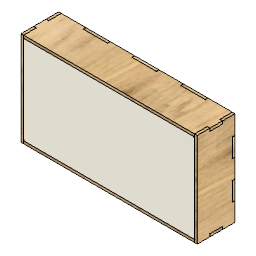
Cronus (Autodesk Fusion 360 design; units mm, degrees)
Autodesk Fusion 360 part; units mm, degrees
note: some values were not read from the file. Set by a fixed rule: which face or edge a step refers to.
(part 1 of 2)
sketch "Sketch1" plane through (0, 0, 0) normal (0, 1, 0) x (1, 0, 0) in component "Display"
  line L0 (0, 0) -> (65.5, 0)
  line L1 (65.5, 0) -> (65.5, -66.5)
  line L2 (65.5, -66.5) -> (0, -66.5)
  line L3 (0, -66.5) -> (0, 0)
  line L4 (0, -66.5) -> (1.55, -66.5) construction
  line L5 (1.55, -66.5) -> (1.55, -65.85) construction
  line L6 (1.55, -65.85) -> (6.55, -65.85)
  line L7 (6.55, -65.85) -> (6.55, -60.85)
  line L8 (6.55, -60.85) -> (1.55, -60.85)
  line L9 (1.55, -60.85) -> (1.55, -65.85)
  line L10 (14.75, -60.85) -> (9.75, -60.85)
  line L11 (9.75, -60.85) -> (9.75, -65.85)
  line L12 (9.75, -65.85) -> (14.75, -65.85)
  line L13 (14.75, -65.85) -> (14.75, -60.85)
  line L14 (22.95, -60.85) -> (17.95, -60.85)
  line L15 (17.95, -60.85) -> (17.95, -65.85)
  line L16 (17.95, -65.85) -> (22.95, -65.85)
  line L17 (22.95, -65.85) -> (22.95, -60.85)
  line L18 (31.15, -60.85) -> (26.15, -60.85)
  line L19 (26.15, -60.85) -> (26.15, -65.85)
  line L20 (26.15, -65.85) -> (31.15, -65.85)
  line L21 (31.15, -65.85) -> (31.15, -60.85)
  line L22 (39.35, -60.85) -> (34.35, -60.85)
  line L23 (34.35, -60.85) -> (34.35, -65.85)
  line L24 (34.35, -65.85) -> (39.35, -65.85)
  line L25 (39.35, -65.85) -> (39.35, -60.85)
  line L26 (47.55, -60.85) -> (42.55, -60.85)
  line L27 (42.55, -60.85) -> (42.55, -65.85)
  line L28 (42.55, -65.85) -> (47.55, -65.85)
  line L29 (47.55, -65.85) -> (47.55, -60.85)
  line L30 (55.75, -60.85) -> (50.75, -60.85)
  line L31 (50.75, -60.85) -> (50.75, -65.85)
  line L32 (50.75, -65.85) -> (55.75, -65.85)
  line L33 (55.75, -65.85) -> (55.75, -60.85)
  line L34 (63.95, -60.85) -> (58.95, -60.85)
  line L35 (58.95, -60.85) -> (58.95, -65.85)
  line L36 (58.95, -65.85) -> (63.95, -65.85)
  line L37 (63.95, -65.85) -> (63.95, -60.85)
  line L38 (6.55, -52.25) -> (1.55, -52.25)
  line L39 (1.55, -52.25) -> (1.55, -57.25)
  line L40 (1.55, -57.25) -> (6.55, -57.25)
  line L41 (6.55, -57.25) -> (6.55, -52.25)
  line L42 (14.75, -52.25) -> (9.75, -52.25)
  line L43 (9.75, -52.25) -> (9.75, -57.25)
  line L44 (9.75, -57.25) -> (14.75, -57.25)
  line L45 (14.75, -57.25) -> (14.75, -52.25)
  line L46 (22.95, -52.25) -> (17.95, -52.25)
  line L47 (17.95, -52.25) -> (17.95, -57.25)
  line L48 (17.95, -57.25) -> (22.95, -57.25)
  line L49 (22.95, -57.25) -> (22.95, -52.25)
  line L50 (31.15, -52.25) -> (26.15, -52.25)
  line L51 (26.15, -52.25) -> (26.15, -57.25)
  line L52 (26.15, -57.25) -> (31.15, -57.25)
  line L53 (31.15, -57.25) -> (31.15, -52.25)
  line L54 (39.35, -52.25) -> (34.35, -52.25)
  line L55 (34.35, -52.25) -> (34.35, -57.25)
  line L56 (34.35, -57.25) -> (39.35, -57.25)
  line L57 (39.35, -57.25) -> (39.35, -52.25)
  line L58 (47.55, -52.25) -> (42.55, -52.25)
  line L59 (42.55, -52.25) -> (42.55, -57.25)
  line L60 (42.55, -57.25) -> (47.55, -57.25)
  line L61 (47.55, -57.25) -> (47.55, -52.25)
  line L62 (55.75, -52.25) -> (50.75, -52.25)
  line L63 (50.75, -52.25) -> (50.75, -57.25)
  line L64 (50.75, -57.25) -> (55.75, -57.25)
  line L65 (55.75, -57.25) -> (55.75, -52.25)
  line L66 (63.95, -52.25) -> (58.95, -52.25)
  line L67 (58.95, -52.25) -> (58.95, -57.25)
  line L68 (58.95, -57.25) -> (63.95, -57.25)
  line L69 (63.95, -57.25) -> (63.95, -52.25)
  line L70 (6.55, -43.65) -> (1.55, -43.65)
  line L71 (1.55, -43.65) -> (1.55, -48.65)
  line L72 (1.55, -48.65) -> (6.55, -48.65)
  line L73 (6.55, -48.65) -> (6.55, -43.65)
  line L74 (14.75, -43.65) -> (9.75, -43.65)
  line L75 (9.75, -43.65) -> (9.75, -48.65)
  line L76 (9.75, -48.65) -> (14.75, -48.65)
  line L77 (14.75, -48.65) -> (14.75, -43.65)
  line L78 (22.95, -43.65) -> (17.95, -43.65)
  line L79 (17.95, -43.65) -> (17.95, -48.65)
  line L80 (17.95, -48.65) -> (22.95, -48.65)
  line L81 (22.95, -48.65) -> (22.95, -43.65)
  line L82 (31.15, -43.65) -> (26.15, -43.65)
  line L83 (26.15, -43.65) -> (26.15, -48.65)
  line L84 (26.15, -48.65) -> (31.15, -48.65)
  line L85 (31.15, -48.65) -> (31.15, -43.65)
  line L86 (39.35, -43.65) -> (34.35, -43.65)
  line L87 (34.35, -43.65) -> (34.35, -48.65)
  line L88 (34.35, -48.65) -> (39.35, -48.65)
  line L89 (39.35, -48.65) -> (39.35, -43.65)
  line L90 (47.55, -43.65) -> (42.55, -43.65)
  line L91 (42.55, -43.65) -> (42.55, -48.65)
  line L92 (42.55, -48.65) -> (47.55, -48.65)
  line L93 (47.55, -48.65) -> (47.55, -43.65)
  line L94 (55.75, -43.65) -> (50.75, -43.65)
  line L95 (50.75, -43.65) -> (50.75, -48.65)
  line L96 (50.75, -48.65) -> (55.75, -48.65)
  line L97 (55.75, -48.65) -> (55.75, -43.65)
  line L98 (63.95, -43.65) -> (58.95, -43.65)
  line L99 (58.95, -43.65) -> (58.95, -48.65)
  line L100 (58.95, -48.65) -> (63.95, -48.65)
  line L101 (63.95, -48.65) -> (63.95, -43.65)
  line L102 (6.55, -35.05) -> (1.55, -35.05)
  line L103 (1.55, -35.05) -> (1.55, -40.05)
  line L104 (1.55, -40.05) -> (6.55, -40.05)
  line L105 (6.55, -40.05) -> (6.55, -35.05)
  line L106 (14.75, -35.05) -> (9.75, -35.05)
  line L107 (9.75, -35.05) -> (9.75, -40.05)
  line L108 (9.75, -40.05) -> (14.75, -40.05)
  line L109 (14.75, -40.05) -> (14.75, -35.05)
  line L110 (22.95, -35.05) -> (17.95, -35.05)
  line L111 (17.95, -35.05) -> (17.95, -40.05)
  line L112 (17.95, -40.05) -> (22.95, -40.05)
  line L113 (22.95, -40.05) -> (22.95, -35.05)
  line L114 (31.15, -35.05) -> (26.15, -35.05)
  line L115 (26.15, -35.05) -> (26.15, -40.05)
  line L116 (26.15, -40.05) -> (31.15, -40.05)
  line L117 (31.15, -40.05) -> (31.15, -35.05)
  line L118 (39.35, -35.05) -> (34.35, -35.05)
  line L119 (34.35, -35.05) -> (34.35, -40.05)
  line L120 (34.35, -40.05) -> (39.35, -40.05)
  line L121 (39.35, -40.05) -> (39.35, -35.05)
  line L122 (47.55, -35.05) -> (42.55, -35.05)
  line L123 (42.55, -35.05) -> (42.55, -40.05)
  line L124 (42.55, -40.05) -> (47.55, -40.05)
  line L125 (47.55, -40.05) -> (47.55, -35.05)
  line L126 (55.75, -35.05) -> (50.75, -35.05)
  line L127 (50.75, -35.05) -> (50.75, -40.05)
  line L128 (50.75, -40.05) -> (55.75, -40.05)
  line L129 (55.75, -40.05) -> (55.75, -35.05)
  line L130 (63.95, -35.05) -> (58.95, -35.05)
  line L131 (58.95, -35.05) -> (58.95, -40.05)
  line L132 (58.95, -40.05) -> (63.95, -40.05)
  line L133 (63.95, -40.05) -> (63.95, -35.05)
  line L134 (6.55, -26.45) -> (1.55, -26.45)
  line L135 (1.55, -26.45) -> (1.55, -31.45)
  line L136 (1.55, -31.45) -> (6.55, -31.45)
  line L137 (6.55, -31.45) -> (6.55, -26.45)
  line L138 (14.75, -26.45) -> (9.75, -26.45)
  line L139 (9.75, -26.45) -> (9.75, -31.45)
  line L140 (9.75, -31.45) -> (14.75, -31.45)
  line L141 (14.75, -31.45) -> (14.75, -26.45)
  line L142 (22.95, -26.45) -> (17.95, -26.45)
  line L143 (17.95, -26.45) -> (17.95, -31.45)
  line L144 (17.95, -31.45) -> (22.95, -31.45)
  line L145 (22.95, -31.45) -> (22.95, -26.45)
  line L146 (31.15, -26.45) -> (26.15, -26.45)
  line L147 (26.15, -26.45) -> (26.15, -31.45)
  line L148 (26.15, -31.45) -> (31.15, -31.45)
  line L149 (31.15, -31.45) -> (31.15, -26.45)
  line L150 (39.35, -26.45) -> (34.35, -26.45)
  line L151 (34.35, -26.45) -> (34.35, -31.45)
  line L152 (34.35, -31.45) -> (39.35, -31.45)
  line L153 (39.35, -31.45) -> (39.35, -26.45)
  line L154 (47.55, -26.45) -> (42.55, -26.45)
  line L155 (42.55, -26.45) -> (42.55, -31.45)
  line L156 (42.55, -31.45) -> (47.55, -31.45)
  line L157 (47.55, -31.45) -> (47.55, -26.45)
  line L158 (55.75, -26.45) -> (50.75, -26.45)
  line L159 (50.75, -26.45) -> (50.75, -31.45)
  line L160 (50.75, -31.45) -> (55.75, -31.45)
  line L161 (55.75, -31.45) -> (55.75, -26.45)
  line L162 (63.95, -26.45) -> (58.95, -26.45)
  line L163 (58.95, -26.45) -> (58.95, -31.45)
  line L164 (58.95, -31.45) -> (63.95, -31.45)
  line L165 (63.95, -31.45) -> (63.95, -26.45)
  line L166 (6.55, -17.85) -> (1.55, -17.85)
  line L167 (1.55, -17.85) -> (1.55, -22.85)
  line L168 (1.55, -22.85) -> (6.55, -22.85)
  line L169 (6.55, -22.85) -> (6.55, -17.85)
  line L170 (14.75, -17.85) -> (9.75, -17.85)
  line L171 (9.75, -17.85) -> (9.75, -22.85)
  line L172 (9.75, -22.85) -> (14.75, -22.85)
  line L173 (14.75, -22.85) -> (14.75, -17.85)
  line L174 (22.95, -17.85) -> (17.95, -17.85)
  line L175 (17.95, -17.85) -> (17.95, -22.85)
  line L176 (17.95, -22.85) -> (22.95, -22.85)
  line L177 (22.95, -22.85) -> (22.95, -17.85)
  line L178 (31.15, -17.85) -> (26.15, -17.85)
  line L179 (26.15, -17.85) -> (26.15, -22.85)
  line L180 (26.15, -22.85) -> (31.15, -22.85)
  line L181 (31.15, -22.85) -> (31.15, -17.85)
  line L182 (39.35, -17.85) -> (34.35, -17.85)
  line L183 (34.35, -17.85) -> (34.35, -22.85)
  line L184 (34.35, -22.85) -> (39.35, -22.85)
  line L185 (39.35, -22.85) -> (39.35, -17.85)
  line L186 (47.55, -17.85) -> (42.55, -17.85)
  line L187 (42.55, -17.85) -> (42.55, -22.85)
  line L188 (42.55, -22.85) -> (47.55, -22.85)
  line L189 (47.55, -22.85) -> (47.55, -17.85)
  line L190 (55.75, -17.85) -> (50.75, -17.85)
  line L191 (50.75, -17.85) -> (50.75, -22.85)
  line L192 (50.75, -22.85) -> (55.75, -22.85)
  line L193 (55.75, -22.85) -> (55.75, -17.85)
  line L194 (63.95, -17.85) -> (58.95, -17.85)
  line L195 (58.95, -17.85) -> (58.95, -22.85)
  line L196 (58.95, -22.85) -> (63.95, -22.85)
  line L197 (63.95, -22.85) -> (63.95, -17.85)
  line L198 (6.55, -9.25) -> (1.55, -9.25)
  line L199 (1.55, -9.25) -> (1.55, -14.25)
  line L200 (1.55, -14.25) -> (6.55, -14.25)
  line L201 (6.55, -14.25) -> (6.55, -9.25)
  line L202 (14.75, -9.25) -> (9.75, -9.25)
  line L203 (9.75, -9.25) -> (9.75, -14.25)
  line L204 (9.75, -14.25) -> (14.75, -14.25)
  line L205 (14.75, -14.25) -> (14.75, -9.25)
  line L206 (22.95, -9.25) -> (17.95, -9.25)
  line L207 (17.95, -9.25) -> (17.95, -14.25)
  line L208 (17.95, -14.25) -> (22.95, -14.25)
  line L209 (22.95, -14.25) -> (22.95, -9.25)
  line L210 (31.15, -9.25) -> (26.15, -9.25)
  line L211 (26.15, -9.25) -> (26.15, -14.25)
  line L212 (26.15, -14.25) -> (31.15, -14.25)
  line L213 (31.15, -14.25) -> (31.15, -9.25)
  line L214 (39.35, -9.25) -> (34.35, -9.25)
  line L215 (34.35, -9.25) -> (34.35, -14.25)
  line L216 (34.35, -14.25) -> (39.35, -14.25)
  line L217 (39.35, -14.25) -> (39.35, -9.25)
  line L218 (47.55, -9.25) -> (42.55, -9.25)
  line L219 (42.55, -9.25) -> (42.55, -14.25)
  line L220 (42.55, -14.25) -> (47.55, -14.25)
  line L221 (47.55, -14.25) -> (47.55, -9.25)
  line L222 (55.75, -9.25) -> (50.75, -9.25)
  line L223 (50.75, -9.25) -> (50.75, -14.25)
  line L224 (50.75, -14.25) -> (55.75, -14.25)
  line L225 (55.75, -14.25) -> (55.75, -9.25)
  line L226 (63.95, -9.25) -> (58.95, -9.25)
  line L227 (58.95, -9.25) -> (58.95, -14.25)
  line L228 (58.95, -14.25) -> (63.95, -14.25)
  line L229 (63.95, -14.25) -> (63.95, -9.25)
  line L230 (6.55, -0.65) -> (1.55, -0.65)
  line L231 (1.55, -0.65) -> (1.55, -5.65)
  line L232 (1.55, -5.65) -> (6.55, -5.65)
  line L233 (6.55, -5.65) -> (6.55, -0.65)
  line L234 (14.75, -0.65) -> (9.75, -0.65)
  line L235 (9.75, -0.65) -> (9.75, -5.65)
  line L236 (9.75, -5.65) -> (14.75, -5.65)
  line L237 (14.75, -5.65) -> (14.75, -0.65)
  line L238 (22.95, -0.65) -> (17.95, -0.65)
  line L239 (17.95, -0.65) -> (17.95, -5.65)
  line L240 (17.95, -5.65) -> (22.95, -5.65)
  line L241 (22.95, -5.65) -> (22.95, -0.65)
  line L242 (31.15, -0.65) -> (26.15, -0.65)
  line L243 (26.15, -0.65) -> (26.15, -5.65)
  line L244 (26.15, -5.65) -> (31.15, -5.65)
  line L245 (31.15, -5.65) -> (31.15, -0.65)
  line L246 (39.35, -0.65) -> (34.35, -0.65)
  line L247 (34.35, -0.65) -> (34.35, -5.65)
  line L248 (34.35, -5.65) -> (39.35, -5.65)
  line L249 (39.35, -5.65) -> (39.35, -0.65)
  line L250 (47.55, -0.65) -> (42.55, -0.65)
  line L251 (42.55, -0.65) -> (42.55, -5.65)
  line L252 (42.55, -5.65) -> (47.55, -5.65)
  line L253 (47.55, -5.65) -> (47.55, -0.65)
  line L254 (55.75, -0.65) -> (50.75, -0.65)
  line L255 (50.75, -0.65) -> (50.75, -5.65)
  line L256 (50.75, -5.65) -> (55.75, -5.65)
  line L257 (55.75, -5.65) -> (55.75, -0.65)
  line L258 (63.95, -0.65) -> (58.95, -0.65)
  line L259 (58.95, -0.65) -> (58.95, -5.65)
  line L260 (58.95, -5.65) -> (63.95, -5.65)
  line L261 (63.95, -5.65) -> (63.95, -0.65)
  line L262 (0, -66.5) -> (1.45, -66.5) construction
  line L263 (32.75, -66.5) -> (32.75, 0) construction
  line L264 (0, -66.5) -> (8, -66.5) construction
  line L265 (8, -66.5) -> (8, 0) construction
  circle A0 centre (8, -33.25) radius 0.95
  circle A1 centre (8, -58.75) radius 0.95 construction
  circle A2 centre (8, -7.75) radius 0.95
  circle A3 centre (57.5, -58.75) radius 0.95
  circle A4 centre (57.5, -33.25) radius 0.95
  circle A5 centre (57.5, -7.75) radius 0.95 construction
  line L266 (0, -66.5) -> (9, -66.5)
  line L267 (9, -66.5) -> (9, -60.85)
  line L268 (9, -60.85) -> (0, -60.85)
  line L269 (0, -60.85) -> (0, -66.5)
  line L270 (65.5, 0) -> (57.5, 0)
  line L271 (56.25, 0) -> (56.25, -5.65)
  line L272 (56.25, -5.65) -> (65.5, -5.65)
  line L273 (65.5, -5.65) -> (65.5, 0)
  dimension "d3" = 65.5
  dimension "d4" = 66.5
  dimension "d5" = 1.55
  dimension "d6" = 0.65
  dimension "d7" = 5
  dimension "d8" = 5
  dimension "d11" = 8.2
  dimension "d12" = 8.6
  dimension "d256" = 8
  dimension "d257" = 1.9
  dimension "d260" = 0
  dimension "d261" = 25.5
  dimension "d276" = 1
  dimension "d277" = 0.5
  constraint horizontal L0
  constraint vertical L1
  constraint horizontal L2
  constraint vertical L3
  constraint coincident L0.start L3.end
  constraint perpendicular L3 L4
  constraint vertical L5
  constraint horizontal L6
  constraint vertical L7
  constraint horizontal L8
  constraint vertical L9
  constraint horizontal L262
  constraint midpoint L2 L263.start
  constraint midpoint L0 L263.end
  constraint horizontal L264
  constraint coincident L0 L265.end
  constraint perpendicular L0 L265
  constraint midpoint L265 A0.centre
  constraint symmetric L263 A0 A4
  constraint symmetric L263 A1 A3
  constraint symmetric L263 A2 A5
  constraint horizontal L266
  constraint vertical L267
  constraint horizontal L268
  constraint vertical L269
  constraint collinear L8 L268
  constraint horizontal L270
  constraint vertical L271
  constraint horizontal L272
  constraint vertical L273
  constraint coincident L271.end L272.start
  constraint coincident L0 L271.start
  constraint collinear L260 L272
  measures "d3" distance of L0.start L0.end
  measures "d4" distance of L0.start L2.end
  measures "d5" distance of L2.end L4.end
  measures "d6" distance of L4.end L5.end
  measures "d7" distance of L5.end L6.end
  measures "d8" distance of L5.end L8.end
  measures "d256" distance of L2.end L264.end
  measures "d257" diameter of A0
  measures "d276" distance of L265 L267
  measures "d277" distance of L257 L271
extrude "Extrude3" add sketch "Sketch1" against normal blind 1.4 contours L0 L1 L2 L3 L8 L260 L267 L268 L271 L272 | L10 L11 L12 L13 | L14 L15 L16 L17 | L18 L19 L20 L21 | L22 L23 L24 L25 | L26 L27 L28 L29 | L30 L31 L32 L33 | L34 L35 L36 L37 | L38 L39 L40 L41 | L42 L43 L44 L45 | L46 L47 L48 L49 | L50 L51 L52 L53 | L54 L55 L56 L57 | L58 L59 L60 L61 | L62 L63 L64 L65 | L66 L67 L68 L69 | L70 L71 L72 L73 | L74 L75 L76 L77 | L78 L79 L80 L81 | L82 L83 L84 L85 | L86 L87 L88 L89 | L90 L91 L92 L93 | L94 L95 L96 L97 | L98 L99 L100 L101 | L102 L103 L104 L105 | L106 L107 L108 L109 | L110 L111 L112 L113 | L114 L115 L116 L117 | L118 L119 L120 L121 | L122 L123 L124 L125 | L126 L127 L128 L129 | L130 L131 L132 L133 | L134 L135 L136 L137 | L138 L139 L140 L141 | L142 L143 L144 L145 | L146 L147 L148 L149 | L150 L151 L152 L153 | L154 L155 L156 L157 | L158 L159 L160 L161 | L162 L163 L164 L165 | L166 L167 L168 L169 | L170 L171 L172 L173 | L174 L175 L176 L177 | L178 L179 L180 L181 | L182 L183 L184 L185 | L186 L187 L188 L189 | L190 L191 L192 L193 | L194 L195 L196 L197 | L198 L199 L200 L201 | L202 L203 L204 L205 | L206 L207 L208 L209 | L210 L211 L212 L213 | L214 L215 L216 L217 | L218 L219 L220 L221 | L222 L223 L224 L225 | L226 L227 L228 L229 | L230 L231 L232 L233 | L234 L235 L236 L237 | L238 L239 L240 L241 | L242 L243 L244 L245 | L246 L247 L248 L249 | L250 L251 L252 L253 | L254 L255 L256 L257 makes body 1 in component "Display"
extrude "Extrude1" add sketch "Sketch1" against normal blind 3 contours L6 L7 L8 L9 L268 | L258 L259 L260 L261 L272 | L10 L11 L12 L13 | L14 L15 L16 L17 | L18 L19 L20 L21 | L22 L23 L24 L25 | L26 L27 L28 L29 | L30 L31 L32 L33 | L34 L35 L36 L37 | L38 L39 L40 L41 | L42 L43 L44 L45 | L46 L47 L48 L49 | L50 L51 L52 L53 | L54 L55 L56 L57 | L58 L59 L60 L61 | L62 L63 L64 L65 | L66 L67 L68 L69 | L70 L71 L72 L73 | L74 L75 L76 L77 | L78 L79 L80 L81 | L82 L83 L84 L85 | L86 L87 L88 L89 | L90 L91 L92 L93 | L94 L95 L96 L97 | L98 L99 L100 L101 | L102 L103 L104 L105 | L106 L107 L108 L109 | L110 L111 L112 L113 | L114 L115 L116 L117 | L118 L119 L120 L121 | L122 L123 L124 L125 | L126 L127 L128 L129 | L130 L131 L132 L133 | L134 L135 L136 L137 | L138 L139 L140 L141 | L142 L143 L144 L145 | L146 L147 L148 L149 | L150 L151 L152 L153 | L154 L155 L156 L157 | L158 L159 L160 L161 | L162 L163 L164 L165 | L166 L167 L168 L169 | L170 L171 L172 L173 | L174 L175 L176 L177 | L178 L179 L180 L181 | L182 L183 L184 L185 | L186 L187 L188 L189 | L190 L191 L192 L193 | L194 L195 L196 L197 | L198 L199 L200 L201 | L202 L203 L204 L205 | L206 L207 L208 L209 | L210 L211 L212 L213 | L214 L215 L216 L217 | L218 L219 L220 L221 | L222 L223 L224 L225 | L226 L227 L228 L229 | L230 L231 L232 L233 | L234 L235 L236 L237 | L238 L239 L240 L241 | L242 L243 L244 L245 | L246 L247 L248 L249 | L250 L251 L252 L253 | L254 L255 L256 L257 bodies 1 in component "Display"
pattern_linear "R-Pattern1" count 4 spacing 65.5 along (1, 0, 0) count 2 spacing 68.5 along (0, 0, 1) of bodies 1 makes body 2 at (90.3041, 0, 51.0047) makes body 3 at (155.8041, 0, 51.0047) makes body 4 at (221.3041, 0, 51.0047) makes body 5 at (24.8041, 0, 119.5047) makes body 6 at (90.3041, 0, 119.5047) makes body 7 at (155.8041, 0, 119.5047) makes body 8 at (221.3041, 0, 119.5047) in component "Display"
sketch "Sketch2" plane through (0, 0, 0) normal (0, 1, 0) x (1, 0, 0) in component "DisplayMount"
  line L0 (262, -135) -> (0, -135)
  line L1 (0, -135) -> (0, 0)
  line L2 (0, 0) -> (262, 0)
  line L3 (262, 0) -> (262, -135)
  line L4 (-1, -136) -> (-1, 1)
  line L5 (-1, 1) -> (263, 1)
  line L6 (263, 1) -> (263, -136)
  line L7 (263, -136) -> (-1, -136)
  point P0 (262, -135)
  constraint horizontal L0
  constraint vertical L1
  constraint horizontal L2
  constraint vertical L3
  constraint coincident L1.end L2.start
  constraint coincident P0 L0.start
extrude "Extrude2" add sketch "Sketch2" along normal blind 3 separate body contours L0 L1 L2 L3 | L4 L5 L6 L7 makes body 9 in component "DisplayMount"
sketch "Sketch3" plane through (0, 3, 0) normal (0, 1, 0) x (-1, 0, 0) in component "DisplayMount"
  line L0 (-263, 136) -> (-263, -1)
  line L1 (-263, -1) -> (1, -1)
  line L2 (1, -1) -> (1, 136)
  line L3 (1, 136) -> (-263, 136)
  circle A0 centre (-57.5, 101.75) radius 0.95
  circle A1 centre (-8, 101.75) radius 0.95
  circle A2 centre (-57.5, 33.25) radius 0.95
  circle A3 centre (-8, 33.25) radius 0.95
  line L4 (-9, 135) -> (0, 135)
  line L5 (0, 135) -> (0, 129.35)
  line L6 (0, 129.35) -> (-9, 129.35)
  line L7 (-9, 129.35) -> (-9, 135)
  line L8 (-65.5, 74.15) -> (-56.25, 74.15)
  line L9 (-56.25, 74.15) -> (-56.25, 68.5)
  line L10 (-56.25, 68.5) -> (-65.5, 68.5)
  line L11 (-65.5, 68.5) -> (-65.5, 74.15)
  line L12 (-9, 66.5) -> (0, 66.5)
  line L13 (0, 66.5) -> (0, 60.85)
  line L14 (0, 60.85) -> (-9, 60.85)
  line L15 (-9, 60.85) -> (-9, 66.5)
  line L16 (-65.5, 5.65) -> (-56.25, 5.65)
  line L17 (-56.25, 5.65) -> (-56.25, 0)
  line L18 (-56.25, 0) -> (-65.5, 0)
  line L19 (-65.5, 0) -> (-65.5, 5.65)
  point P0 (-9, 135)
  point P1 (0, 129.35)
  point P2 (-9, 66.5)
  point P3 (0, 60.85)
  point P4 (-65.5, 74.15)
  point P5 (-56.25, 68.5)
  point P6 (-65.5, 5.65)
  point P7 (-56.25, 0)
  constraint horizontal L4
  constraint vertical L5
  constraint horizontal L6
  constraint vertical L7
  constraint horizontal L8
  constraint vertical L9
  constraint horizontal L10
  constraint vertical L11
  constraint horizontal L12
  constraint vertical L13
  constraint horizontal L14
  constraint vertical L15
  constraint horizontal L16
  constraint vertical L17
  constraint horizontal L18
  constraint vertical L19
  constraint coincident P2 L12.start
  constraint coincident P3 L13.end
  constraint coincident P0 L4.start
  constraint coincident P1 L5.end
  constraint coincident P4 L8.start
  constraint coincident P5 L9.end
  constraint coincident P6 L16.start
  constraint coincident P7 L17.end
extrude "Extrude3'" cut sketch "Sketch3" against normal up to surface (3 mm away) contours A0 | A1 | A2 | A3 | L4 L5 L6 L7 | L8 L9 L10 L11 | L12 L13 L14 L15 | L16 L17 L18 L19 bodies 9 in component "DisplayMount"
pattern_linear "R-Pattern3" count 4 spacing 65.5 along (1, 0, 0) of "Extrude3'" in component "DisplayMount"
ref_plane "WorkPlane1" through (131, 10, 67.5) normal (0, 1, 0) x (0, 0, 1) in component "PowerSupply"
sketch "Sketch2 (2)" plane through (0, 10, 0) normal (0, 1, 0) x (1, 0, 0) in component "PowerSupply"
  line L0 (236, -116) -> (178, -116)
  line L1 (178, -116) -> (178, -31)
  line L2 (178, -31) -> (236, -31)
  line L3 (236, -31) -> (236, -116)
  line L4 (236, -116) -> (230, -116) construction
  line L5 (230, -116) -> (230, -113) construction
  circle A0 centre (230, -113) radius 1.25
  line L6 (230, -113) -> (183, -113) construction
  line L7 (183, -113) -> (183, -35) construction
  line L8 (183, -35) -> (230, -35) construction
  line L9 (230, -35) -> (230, -113) construction
  circle A1 centre (183, -35) radius 1.25
  line L10 (230, -113) -> (183, -113) construction
  line L11 (183, -113) -> (183, -35) construction
  line L12 (183, -35) -> (230, -35) construction
  line L13 (230, -35) -> (230, -113) construction
  line L14 (230, -113) -> (183, -113) construction
  line L15 (183, -113) -> (183, -35) construction
  line L16 (183, -35) -> (230, -35) construction
  line L17 (230, -35) -> (230, -113) construction
  circle A2 centre (183, -113) radius 1.25
  circle A3 centre (230, -35) radius 1.25
  dimension "d145" = 58
  dimension "d146" = 85
  dimension "d147" = 6
  dimension "d148" = 90
  dimension "d149" = 3
  dimension "d150" = 2.5
  dimension "d151" = 47
  dimension "d152" = 78
  dimension "d153" = 2.5
  dimension "d242" = 2.5
  dimension "d243" = 2.5
  constraint horizontal L0
  constraint vertical L1
  constraint horizontal L2
  constraint vertical L3
  constraint coincident L0 L4.end
  constraint coincident L5.end A0.centre
  constraint horizontal L6
  constraint vertical L7
  constraint horizontal L8
  constraint vertical L9
  constraint coincident L7.end L8.start
  constraint horizontal L10
  constraint vertical L11
  constraint horizontal L12
  constraint vertical L13
  constraint horizontal L14
  constraint vertical L15
  constraint horizontal L16
  constraint vertical L17
  constraint coincident L6.end L7.start
  constraint coincident L8.end L9.start
  measures "d145" distance of L0.start L0.end
  measures "d146" distance of L0.start L2.end
  measures "d147" distance of L0.start L4.end
  measures "d148" angle of L4 L5
  measures "d149" distance of L4.end L5.end
  measures "d150" diameter of A0
  measures "d151" distance of L5.end L6.end
  measures "d152" distance of L5.end L8.end
  measures "d153" diameter of A1
  measures "d242" diameter of A2
  measures "d243" diameter of A3
extrude "Extrude1'" add sketch "Sketch2 (2)" along normal blind 34 separate body makes body 10 in component "PowerSupply"
sketch "Sketch11" plane through (0, 3, 0) normal (0, 1, 0) x (-1, 0, 0) in component "DisplayMount"
  line L0 (1, 136) -> (-263, 136)
  line L1 (-263, 136) -> (-263, -1)
  line L2 (-263, -1) -> (1, -1)
  circle A0 centre (-230, 113) radius 1.25
  circle A1 centre (-183, 35) radius 1.25
  circle A2 centre (-230, 113) radius 3.5
  circle A3 centre (-183, 35) radius 3.5
  line L3 (1, -1) -> (1, 136)
  line L4 (-97.9526, 89.8787) -> (-31.9526, 89.8787) construction
  line L5 (-31.9526, 89.8787) -> (-31.9526, 43.8787) construction
  line L6 (-31.9526, 43.8787) -> (-97.9526, 43.8787) construction
  line L7 (-97.9526, 43.8787) -> (-97.9526, 89.8787) construction
  circle A4 centre (-97.9526, 89.8787) radius 1
  circle A5 centre (-31.9526, 89.8787) radius 1
  circle A6 centre (-97.9526, 43.8787) radius 1
  circle A7 centre (-31.9526, 43.8787) radius 1
  circle A8 centre (-97.9526, 89.8787) radius 2.5
  circle A9 centre (-31.9526, 89.8787) radius 2.5
  circle A10 centre (-31.9526, 43.8787) radius 2.5
  circle A11 centre (-97.9526, 43.8787) radius 2.5
  circle A12 centre (-183, 113) radius 1.25
  circle A13 centre (-230, 35) radius 1.25
  circle A14 centre (-183, 113) radius 3.5
  circle A15 centre (-230, 35) radius 3.5
  circle A16 centre (-254, 33.25) radius 0.95
  line L8 (-262, 68.5) -> (-262, 74.15)
  line L9 (-262, 74.15) -> (-252.75, 74.15)
  line L10 (-252.75, 74.15) -> (-252.75, 68.5)
  line L11 (-252.75, 68.5) -> (-262, 68.5)
  line L12 (-205.5, 129.35) -> (-205.5, 135)
  line L13 (-205.5, 135) -> (-196.5, 135)
  line L14 (-196.5, 135) -> (-196.5, 129.35)
  line L15 (-196.5, 129.35) -> (-205.5, 129.35)
  circle A17 centre (-204.5, 101.75) radius 0.95
  circle A18 centre (-204.5, 33.25) radius 0.95
  line L16 (-262, 0) -> (-262, 5.65)
  line L17 (-262, 5.65) -> (-252.75, 5.65)
  line L18 (-252.75, 5.65) -> (-252.75, 0)
  line L19 (-252.75, 0) -> (-262, 0)
  line L20 (-205.5, 60.85) -> (-205.5, 66.5)
  line L21 (-205.5, 66.5) -> (-196.5, 66.5)
  line L22 (-196.5, 66.5) -> (-196.5, 60.85)
  line L23 (-196.5, 60.85) -> (-205.5, 60.85)
  circle A19 centre (-254, 101.75) radius 0.95
  circle A20 centre (-188.5, 33.25) radius 0.95
  line L24 (-196.5, 68.5) -> (-196.5, 74.15)
  line L25 (-196.5, 74.15) -> (-187.25, 74.15)
  line L26 (-187.25, 74.15) -> (-187.25, 68.5)
  line L27 (-187.25, 68.5) -> (-196.5, 68.5)
  line L28 (-140, 129.35) -> (-140, 135)
  line L29 (-140, 135) -> (-131, 135)
  line L30 (-131, 135) -> (-131, 129.35)
  line L31 (-131, 129.35) -> (-140, 129.35)
  circle A21 centre (-139, 101.75) radius 0.95
  circle A22 centre (-139, 33.25) radius 0.95
  line L32 (-196.5, 0) -> (-196.5, 5.65)
  line L33 (-196.5, 5.65) -> (-187.25, 5.65)
  line L34 (-187.25, 5.65) -> (-187.25, 0)
  line L35 (-187.25, 0) -> (-196.5, 0)
  line L36 (-140, 60.85) -> (-140, 66.5)
  line L37 (-140, 66.5) -> (-131, 66.5)
  line L38 (-131, 66.5) -> (-131, 60.85)
  line L39 (-131, 60.85) -> (-140, 60.85)
  circle A23 centre (-188.5, 101.75) radius 0.95
  circle A24 centre (-123, 33.25) radius 0.95
  line L40 (-131, 68.5) -> (-131, 74.15)
  line L41 (-131, 74.15) -> (-121.75, 74.15)
  line L42 (-121.75, 74.15) -> (-121.75, 68.5)
  line L43 (-121.75, 68.5) -> (-131, 68.5)
  line L44 (-74.5, 129.35) -> (-74.5, 135)
  line L45 (-74.5, 135) -> (-65.5, 135)
  line L46 (-65.5, 135) -> (-65.5, 129.35)
  line L47 (-65.5, 129.35) -> (-74.5, 129.35)
  circle A25 centre (-73.5, 101.75) radius 0.95
  circle A26 centre (-73.5, 33.25) radius 0.95
  line L48 (-131, 0) -> (-131, 5.65)
  line L49 (-131, 5.65) -> (-121.75, 5.65)
  line L50 (-121.75, 5.65) -> (-121.75, 0)
  line L51 (-121.75, 0) -> (-131, 0)
  line L52 (-74.5, 60.85) -> (-74.5, 66.5)
  line L53 (-74.5, 66.5) -> (-65.5, 66.5)
  line L54 (-65.5, 66.5) -> (-65.5, 60.85)
  line L55 (-65.5, 60.85) -> (-74.5, 60.85)
  circle A27 centre (-123, 101.75) radius 0.95
  circle A28 centre (-57.5, 33.25) radius 0.95
  line L56 (-65.5, 68.5) -> (-65.5, 74.15)
  line L57 (-65.5, 74.15) -> (-56.25, 74.15)
  line L58 (-56.25, 74.15) -> (-56.25, 68.5)
  line L59 (-56.25, 68.5) -> (-65.5, 68.5)
  line L60 (-9, 129.35) -> (-9, 135)
  line L61 (-9, 135) -> (0, 135)
  line L62 (0, 135) -> (0, 129.35)
  line L63 (0, 129.35) -> (-9, 129.35)
  circle A29 centre (-8, 101.75) radius 0.95
  circle A30 centre (-8, 33.25) radius 0.95
  line L64 (-65.5, 0) -> (-65.5, 5.65)
  line L65 (-65.5, 5.65) -> (-56.25, 5.65)
  line L66 (-56.25, 5.65) -> (-56.25, 0)
  line L67 (-56.25, 0) -> (-65.5, 0)
  line L68 (-9, 60.85) -> (-9, 66.5)
  line L69 (-9, 66.5) -> (0, 66.5)
  line L70 (0, 66.5) -> (0, 60.85)
  line L71 (0, 60.85) -> (-9, 60.85)
  circle A31 centre (-57.5, 101.75) radius 0.95
  dimension "d156" = 7
  dimension "d157" = 7
  dimension "d166" = 66
  dimension "d167" = 46
  dimension "d168" = 2
  dimension "d169" = 2
  dimension "d170" = 2
  dimension "d171" = 2
  dimension "d172" = 5
  dimension "d173" = 5
  dimension "d174" = 5
  dimension "d175" = 5
  dimension "d244" = 7
  dimension "d245" = 7
  constraint concentric A0 A2
  constraint concentric A1 A3
  constraint horizontal L4
  constraint vertical L5
  constraint horizontal L6
  constraint vertical L7
  constraint coincident L4.start L7.end
  constraint coincident L4.end L5.start
  constraint coincident L6.end L7.start
  constraint coincident L5.end L6.start
  constraint concentric A4 A8
  constraint concentric A5 A9
  constraint concentric A7 A10
  constraint concentric A6 A11
  constraint concentric A12 A14
  constraint concentric A13 A15
  measures "d156" diameter of A2
  measures "d157" diameter of A3
  measures "d166" distance of L4.start L4.end
  measures "d167" distance of L4.start L6.end
  measures "d168" diameter of A4
  measures "d169" diameter of A5
  measures "d170" diameter of A6
  measures "d171" diameter of A7
  measures "d172" diameter of A8
  measures "d173" diameter of A9
  measures "d174" diameter of A10
  measures "d175" diameter of A11
  measures "d244" diameter of A14
  measures "d245" diameter of A15
extrude "Extrude17" add sketch "Sketch11" along normal up to surface (7 mm away) contours A2 | A3 | A8 | A9 | A10 | A11 | A14 | A15 bodies 9 in component "DisplayMount"
chamfer "Chamfer4" distance 3 angle 45 8 edges at (233.2631, 3, 114.2657) (186.2631, 3, 114.2657) (233.2631, 3, 36.2657) (186.2631, 3, 36.2657) (100.2835, 3, 44.7827) (34.2835, 3, 44.7827) (100.2835, 3, 90.7827) (34.2835, 3, 90.7827) on bodies 9 in component "DisplayMount"
sketch "Sketch4" plane through (0, 3, 0) normal (0, 1, 0) x (-1, 0, 0) in component "DisplayMount"
  line L0 (-263, 136) -> (-263, -1)
  line L1 (-263, -1) -> (1, -1)
  line L2 (1, -1) -> (1, 136)
  line L3 (1, 136) -> (-263, 136)
  line L4 (-131, 136) -> (-131, -1) construction
  line L5 (-131, 136) -> (1, 136) construction
  line L6 (-65, 136) -> (-131, 136) construction
  line L7 (-65, 136) -> (1, 136) construction
  line L8 (-98, 136) -> (-98, -1) construction
  line L9 (-32, 136) -> (-32, -1) construction
  line L10 (-263, 67.5) -> (1, 67.5) construction
  line L11 (-108, 136) -> (-88, 136)
  line L12 (-88, 136) -> (-88, 133)
  line L13 (-88, 133) -> (-108, 133)
  line L14 (-108, 133) -> (-108, 136)
  line L15 (-42, 136) -> (-22, 136)
  line L16 (-22, 136) -> (-22, 133)
  line L17 (-22, 133) -> (-42, 133)
  line L18 (-42, 133) -> (-42, 136)
  circle A0 centre (-98, 133) radius 3
  circle A1 centre (-32, 133) radius 3
  circle A2 centre (-98, 133) radius 1.6
  circle A3 centre (-32, 133) radius 1.6
  line L19 (-22, -1) -> (-22, 2)
  line L20 (-42, 2) -> (-42, -1)
  circle A4 centre (-32, 2) radius 3
  line L21 (-42, -1) -> (-22, -1)
  line L22 (-22, 2) -> (-42, 2)
  circle A5 centre (-32, 2) radius 1.6
  circle A6 centre (-98, 2) radius 3
  circle A7 centre (-98, 2) radius 1.6
  line L23 (-108, 2) -> (-108, -1)
  line L24 (-88, 2) -> (-108, 2)
  line L25 (-88, -1) -> (-88, 2)
  line L26 (-108, -1) -> (-88, -1)
  line L27 (-240, 2) -> (-220, 2)
  line L28 (-240, 136) -> (-240, 133)
  circle A8 centre (-230, 2) radius 1.6
  line L29 (-240, 133) -> (-220, 133)
  line L30 (-220, 2) -> (-220, -1)
  circle A9 centre (-230, 133) radius 3
  line L31 (-240, -1) -> (-240, 2)
  circle A10 centre (-230, 2) radius 3
  line L32 (-220, 136) -> (-240, 136)
  circle A11 centre (-230, 133) radius 1.6
  line L33 (-220, 133) -> (-220, 136)
  line L34 (-220, -1) -> (-240, -1)
  line L35 (-154, 2) -> (-154, -1)
  circle A12 centre (-164, 2) radius 3
  circle A13 centre (-164, 133) radius 3
  circle A14 centre (-164, 2) radius 1.6
  line L36 (-174, 133) -> (-154, 133)
  line L37 (-174, 136) -> (-174, 133)
  line L38 (-154, -1) -> (-174, -1)
  line L39 (-154, 133) -> (-154, 136)
  circle A15 centre (-164, 133) radius 1.6
  line L40 (-174, -1) -> (-174, 2)
  line L41 (-154, 136) -> (-174, 136)
  line L42 (-174, 2) -> (-154, 2)
  circle A16 centre (-254, 33.25) radius 0.95
  line L43 (-262, 68.5) -> (-262, 74.15)
  line L44 (-262, 74.15) -> (-252.75, 74.15)
  line L45 (-252.75, 74.15) -> (-252.75, 68.5)
  line L46 (-252.75, 68.5) -> (-262, 68.5)
  line L47 (-205.5, 129.35) -> (-205.5, 135)
  line L48 (-205.5, 135) -> (-196.5, 135)
  line L49 (-196.5, 135) -> (-196.5, 129.35)
  line L50 (-196.5, 129.35) -> (-205.5, 129.35)
  circle A17 centre (-204.5, 101.75) radius 0.95
  circle A18 centre (-204.5, 33.25) radius 0.95
  line L51 (-262, 0) -> (-262, 5.65)
  line L52 (-262, 5.65) -> (-252.75, 5.65)
  line L53 (-252.75, 5.65) -> (-252.75, 0)
  line L54 (-252.75, 0) -> (-262, 0)
  line L55 (-205.5, 60.85) -> (-205.5, 66.5)
  line L56 (-205.5, 66.5) -> (-196.5, 66.5)
  line L57 (-196.5, 66.5) -> (-196.5, 60.85)
  line L58 (-196.5, 60.85) -> (-205.5, 60.85)
  circle A19 centre (-254, 101.75) radius 0.95
  line L59 (-196.5, 68.5) -> (-196.5, 74.15)
  line L60 (-196.5, 74.15) -> (-187.25, 74.15)
  line L61 (-187.25, 74.15) -> (-187.25, 68.5)
  line L62 (-187.25, 68.5) -> (-196.5, 68.5)
  line L63 (-140, 129.35) -> (-140, 135)
  line L64 (-140, 135) -> (-131, 135)
  line L65 (-131, 135) -> (-131, 129.35)
  line L66 (-131, 129.35) -> (-140, 129.35)
  circle A20 centre (-139, 101.75) radius 0.95
  circle A21 centre (-139, 33.25) radius 0.95
  line L67 (-196.5, 0) -> (-196.5, 5.65)
  line L68 (-196.5, 5.65) -> (-187.25, 5.65)
  line L69 (-187.25, 5.65) -> (-187.25, 0)
  line L70 (-187.25, 0) -> (-196.5, 0)
  line L71 (-140, 60.85) -> (-140, 66.5)
  line L72 (-140, 66.5) -> (-131, 66.5)
  line L73 (-131, 66.5) -> (-131, 60.85)
  line L74 (-131, 60.85) -> (-140, 60.85)
  circle A22 centre (-188.5, 101.75) radius 0.95
  circle A23 centre (-123, 33.25) radius 0.95
  line L75 (-131, 68.5) -> (-131, 74.15)
  line L76 (-131, 74.15) -> (-121.75, 74.15)
  line L77 (-121.75, 74.15) -> (-121.75, 68.5)
  line L78 (-121.75, 68.5) -> (-131, 68.5)
  line L79 (-74.5, 129.35) -> (-74.5, 135)
  line L80 (-74.5, 135) -> (-65.5, 135)
  line L81 (-65.5, 135) -> (-65.5, 129.35)
  line L82 (-65.5, 129.35) -> (-74.5, 129.35)
  circle A24 centre (-73.5, 101.75) radius 0.95
  circle A25 centre (-73.5, 33.25) radius 0.95
  line L83 (-131, 0) -> (-131, 5.65)
  line L84 (-131, 5.65) -> (-121.75, 5.65)
  line L85 (-121.75, 5.65) -> (-121.75, 0)
  line L86 (-121.75, 0) -> (-131, 0)
  line L87 (-74.5, 60.85) -> (-74.5, 66.5)
  line L88 (-74.5, 66.5) -> (-65.5, 66.5)
  line L89 (-65.5, 66.5) -> (-65.5, 60.85)
  line L90 (-65.5, 60.85) -> (-74.5, 60.85)
  circle A26 centre (-123, 101.75) radius 0.95
  circle A27 centre (-57.5, 33.25) radius 0.95
  line L91 (-65.5, 68.5) -> (-65.5, 74.15)
  line L92 (-65.5, 74.15) -> (-56.25, 74.15)
  line L93 (-56.25, 74.15) -> (-56.25, 68.5)
  line L94 (-56.25, 68.5) -> (-65.5, 68.5)
  line L95 (-9, 129.35) -> (-9, 135)
  line L96 (-9, 135) -> (0, 135)
  line L97 (0, 135) -> (0, 129.35)
  line L98 (0, 129.35) -> (-9, 129.35)
  circle A28 centre (-8, 101.75) radius 0.95
  circle A29 centre (-8, 33.25) radius 0.95
  line L99 (-65.5, 0) -> (-65.5, 5.65)
  line L100 (-65.5, 5.65) -> (-56.25, 5.65)
  line L101 (-56.25, 5.65) -> (-56.25, 0)
  line L102 (-56.25, 0) -> (-65.5, 0)
  line L103 (-9, 60.85) -> (-9, 66.5)
  line L104 (-9, 66.5) -> (0, 66.5)
  line L105 (0, 66.5) -> (0, 60.85)
  line L106 (0, 60.85) -> (-9, 60.85)
  circle A30 centre (-57.5, 101.75) radius 0.95
  line L107 (-263, 114.25) -> (-260, 114.25)
  line L108 (-260, 114.25) -> (-260, 89.25)
  line L109 (-260, 89.25) -> (-263, 89.25)
  line L110 (-263, 89.25) -> (-263, 114.25)
  circle A31 centre (-260, 101.75) radius 1.6
  circle A32 centre (-260, 101.75) radius 3
  circle A33 centre (-97.9526, 89.8787) radius 5.5
  circle A34 centre (-97.9526, 43.8787) radius 5.5
  arc A35 (-188.9673, 32.4229) -> (-189.3593, 33.655) centre (-183, 35) ccw
  arc A36 (-189.3593, 33.655) -> (-188.9673, 32.4229) centre (-188.5, 33.25) ccw
  circle A37 centre (-183, 113) radius 6.5
  circle A38 centre (-230, 113) radius 6.5
  circle A39 centre (-230, 35) radius 6.5
  circle A40 centre (-31.9526, 43.8787) radius 5.5
  circle A41 centre (-31.9526, 89.8787) radius 5.5
  line L111 (-254, 101.75) -> (-263, 101.75) construction
  line L112 (-263, 20.75) -> (-260, 20.75)
  line L113 (-263, 45.75) -> (-263, 20.75)
  line L114 (-260, 20.75) -> (-260, 45.75)
  circle A42 centre (-260, 33.25) radius 1.6
  circle A43 centre (-260, 33.25) radius 3
  line L115 (-260, 45.75) -> (-263, 45.75)
  line L116 (1, 114.25) -> (-2, 114.25)
  line L117 (1, 89.25) -> (1, 114.25)
  line L118 (-2, 114.25) -> (-2, 89.25)
  circle A44 centre (-2, 101.75) radius 3
  circle A45 centre (-2, 101.75) radius 1.6
  line L119 (-2, 89.25) -> (1, 89.25)
  line L120 (-2, 45.75) -> (1, 45.75)
  line L121 (1, 45.75) -> (1, 20.75)
  line L122 (-2, 20.75) -> (-2, 45.75)
  circle A46 centre (-2, 33.25) radius 1.6
  circle A47 centre (-2, 33.25) radius 3
  line L123 (1, 20.75) -> (-2, 20.75)
  point P0 (-32, -1)
  point P1 (-98, -1)
  point P2 (-230, 136)
  point P3 (-230, -1)
  point P4 (-230, -1)
  point P5 (-164, 136)
  point P6 (-164, -1)
  point P7 (-164, -1)
  dimension "d72" = 20
  dimension "d73" = 3
  dimension "d74" = 20
  dimension "d75" = 3
  dimension "d76" = 6
  dimension "d77" = 6
  dimension "d78" = 3.2
  dimension "d79" = 3.2
  dimension "d268" = 3
  dimension "d269" = 3.2
  dimension "d270" = 6
  dimension "d290" = 25
  constraint midpoint L3 L4.start
  constraint midpoint L1 L4.end
  constraint coincident L2.end L3.start
  constraint midpoint L5 L6.start
  constraint midpoint L6 L8.start
  constraint coincident L1 P1
  constraint perpendicular L1 L8
  constraint midpoint L7 L9.start
  constraint coincident L1 P0
  constraint perpendicular L1 L9
  constraint midpoint L0 L10.start
  constraint midpoint L2 L10.end
  constraint horizontal L11
  constraint vertical L12
  constraint horizontal L13
  constraint vertical L14
  constraint midpoint L6 L11
  constraint horizontal L15
  constraint vertical L16
  constraint horizontal L17
  constraint vertical L18
  constraint midpoint L7 L15
  constraint midpoint L13 A0.centre
  constraint midpoint L17 A1.centre
  constraint concentric A0 A2
  constraint concentric A1 A3
  constraint symmetric L8.start L10 P1
  constraint symmetric L9.start L10 P0
  constraint symmetric L10 L11.start L23.end
  constraint symmetric L10 L11.end L25.start
  constraint symmetric L10 L12.end L24.start
  constraint symmetric L10 L13.end L23.start
  constraint symmetric L10 L15.start L20.end
  constraint symmetric L10 L15.end L19.start
  constraint symmetric L10 L16.end L19.end
  constraint symmetric L10 L17.end L20.start
  constraint symmetric L10 A0 A6
  constraint symmetric L10 A1 A4
  constraint symmetric L10 A2 A7
  constraint symmetric L10 A3 A5
  constraint symmetric L4 L9.start P2
  constraint symmetric L4 P0 P4
  constraint symmetric L4 L15.start L32.start
  constraint symmetric L4 L15.end L28.start
  constraint symmetric L4 L16.end L28.end
  constraint symmetric L4 L17.end L29.end
  constraint symmetric L4 A1 A9
  constraint symmetric L4 A3 A11
  constraint symmetric L4 L19.start L31.start
  constraint symmetric L4 L19.end L27.start
  constraint symmetric L4 L20.end L30.end
  constraint symmetric L4 L20.start L27.end
  constraint symmetric L4 A4 A10
  constraint symmetric L4 A5 A8
  constraint symmetric L4 L8.start P5
  constraint symmetric L4 P1 P7
  constraint symmetric L4 L11.start L39.end
  constraint symmetric L4 L11.end L37.start
  constraint symmetric L4 L12.end L36.start
  constraint symmetric L4 L13.end L36.end
  constraint symmetric L4 A0 A13
  constraint symmetric L4 A2 A15
  constraint symmetric L4 L23.start L35.start
  constraint symmetric L4 L24.start L40.end
  constraint symmetric L4 L23.end L35.end
  constraint symmetric L4 L25.start L38.end
  constraint symmetric L4 A6 A12
  constraint symmetric L4 A7 A14
  constraint coincident L0 L107.start
  constraint horizontal L107
  constraint vertical L108
  constraint horizontal L109
  constraint vertical L110
  constraint midpoint L108 A31.centre
  constraint concentric A31 A32
  constraint coincident A19.centre L111.start
  constraint coincident L0 L111.end
  constraint perpendicular L0 L111
  constraint coincident A31.centre L111
  constraint symmetric L10 L107.start L112.start
  constraint symmetric L10 L107.end L112.end
  constraint symmetric L10 L108.end L114.end
  constraint symmetric L10 L109.end L113.start
  constraint symmetric L10 A31 A42
  constraint symmetric L10 A32 A43
  constraint symmetric L4 L107.start L116.start
  constraint symmetric L4 L107.end L116.end
  constraint symmetric L4 L108.end L118.end
  constraint symmetric L4 L109.end L117.start
  constraint symmetric L4 A31 A45
  constraint symmetric L4 A32 A44
  constraint symmetric L4 L112.start L121.end
  constraint symmetric L4 L112.end L122.start
  constraint symmetric L4 L113.start L120.end
  constraint symmetric L4 L114.end L120.start
  constraint symmetric L4 A42 A46
  constraint symmetric L4 A43 A47
  measures "d72" distance of L11.start L11.end
  measures "d73" distance of L11.start L13.end
  measures "d74" distance of L15.start L15.end
  measures "d75" distance of L15.start L17.end
  measures "d76" diameter of A0
  measures "d77" diameter of A1
  measures "d78" diameter of A2
  measures "d79" diameter of A3
  measures "d268" distance of L107.start L107.end
  measures "d269" diameter of A31
  measures "d270" diameter of A32
  measures "d290" distance of L107 L109
extrude "Extrude4" add sketch "Sketch4" along normal up to surface (46 mm away) contours L0 L107 L108 L110 A32 | L3 L28 L29 A9 L32 | L0 L108 L109 L110 A32 | L108 A31 A32 | L3 L29 A9 L32 L33 | L29 A9 A11 | L108 A31 A32 | L29 A9 A11 | L0 L113 L114 A43 L115 | L3 A13 L36 L37 L41 | L0 L112 L113 L114 A43 | L114 A42 A43 | L3 A13 L36 L39 L41 | A13 L36 A15 | L114 A42 A43 | A13 L36 A15 | L3 L11 L13 L14 A0 | L1 L27 L31 A10 L34 | L3 L11 L12 L13 A0 | L13 A0 A2 | L1 L27 L30 A10 L34 | L27 A8 A10 | L13 A0 A2 | L27 A8 A10 | L3 L15 L17 L18 A1 | L1 A12 L38 L40 L42 | L3 L15 L16 L17 A1 | L17 A1 A3 | L1 L35 A12 L38 L42 | A12 A14 L42 | L17 A1 A3 | A12 A14 L42 | L1 A6 L23 L24 L26 | L2 L116 L117 L118 A44 | L1 A6 L24 L25 L26 | A6 A7 L24 | L118 A44 A45 | L2 L117 L118 A44 L119 | A6 A7 L24 | L118 A44 A45 | L1 L20 A4 L21 L22 | L2 L120 L121 L122 A47 | L1 L19 A4 L21 L22 | A4 L22 A5 | L122 A46 A47 | L2 L121 L122 A47 L123 | A4 L22 A5 | L122 A46 A47 bodies 9 in component "DisplayMount"